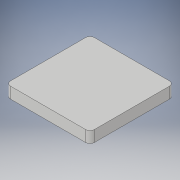
# Autodesk Inventor part: Marco - Asiento Triciclo
Saved by Autodesk Inventor 2019 (Build 230136000, 136)
## iProperties
Created: 2019-11-15
Part Number: Marco - Asiento Triciclo
Material: Genérico
Document SubType Name: Modeling
Designer: eddysanoli
Density: 1 g/cm^3
Appearance: Valor por defecto
Author: eddysanoli
Autodesk Inventor part; units mm, degrees
ref_plane "YZ Plane" through (0, 0, 0) normal (1, 0, 0) x (0, 1, 0)
ref_plane "XZ Plane" through (0, 0, 0) normal (0, 1, 0) x (-1, 0, 0)
ref_plane "XY Plane" through (0, 0, 0) normal (0, 0, 1) x (1, 0, 0)
sketch "Boceto1" plane through (0, 0, 0) normal (0, 1, 0) x (-1, 0, 0)
  line L0 (4, 0) -> (71, 0)
  line L1 (75, -4) -> (75, -71)
  line L2 (71, -75) -> (4, -75)
  line L3 (0, -71) -> (0, -4)
  arc A0 (75, -4) -> (71, 0) centre (71, -4) ccw
  arc A1 (71, -75) -> (75, -71) centre (71, -71) ccw
  arc A2 (0, -71) -> (4, -75) centre (4, -71) ccw
  arc A3 (4, 0) -> (0, -4) centre (4, -4) ccw
  point P0 (0, 0)
  point P1 (75, 0)
  dimension "d0" = 75
  dimension "d1" = 4
  constraints: 8 end point, 8 point on circle, 8 tangent, 4 centre point, 4 point on line, 3 equal radius, 2 parallel, 2 perpendicular, 1 horizontal
  measures "d0" distance of point (0, 0) point (75, 0)
  measures "d1" radius of A0
extrude "Extrusión1" add sketch "Boceto1" along normal blind 10
